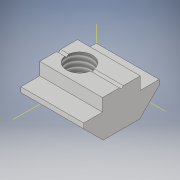
# Autodesk Inventor part: BTwnikel2_trajan20_21
Saved by Autodesk Inventor 2022.2 (Build 262287000, 287)
## iProperties
Company: HTBLA Kaindorf
RuleStatus: InUse
Created: 2022-06-22
Part Number: BTwnikel2_trajan20_21
Project: Zeichenmaschine_v2
Material: Generisch
Description: nutenstein
Document SubType Name: Modeling
Designer: trajan20
Density: 1 g/cm^3
Appearance: Vorgabe
Mass: 0.412179 g
Surface Area: 4.70943 cm^2
Volume: 0.412179 cm^3
AfterDocNew0: iProperties-Editor_aufrufen
Author: jan
Keywords: 2021
Autodesk Inventor part; units mm, degrees
ref_plane "YZ Plane" through (0, 0, 0) normal (1, 0, 0) x (0, 1, 0)
ref_plane "XZ Plane" through (0, 0, 0) normal (0, 1, 0) x (-1, 0, 0)
ref_plane "XY Plane" through (0, 0, 0) normal (0, 0, 1) x (1, 0, 0)
sketch "Skizze3" plane through (0, 0, 0) normal (0, 1, 0) x (-1, 0, 0)
  line L0 (0, 3.9) -> (-3, 3.9)
  line L1 (-3, 3.9) -> (-3, 5.9)
  line L2 (0, 3.9) -> (0, 3.1)
  line L3 (0, 3.1) -> (-3.1, 0)
  line L4 (-3, 5.9) -> (-5.7, 5.9)
  line L5 (-5.7, 5.9) -> (-6, 5.6)
  line L6 (-6, 5.6) -> (-6, 0)
  line L7 (-6, 0) -> (-3.1, 0)
  point P0 (0, 0)
  dimension "d6" = 3
  dimension "d7" = 6
  dimension "d8" = 3.1
  dimension "d9" = 5.9
  dimension "d10" = 135
  dimension "d11" = 0.3
  dimension "d12" = 2
  dimension "d13" = 135
  constraints: 16 end point, 3 perpendicular, 2 horizontal, 2 point on line, 1 vertical
  measures "d6" distance between parallel lines of L6 L1
  measures "d7" distance between parallel lines of L2 L6
  measures "d8" distance from line of L7 L2.end
  measures "d9" distance between parallel lines of L4 L7
  measures "d10" angle of L6 L5
  measures "d11" horizontal distance of L4.end L5.end
  measures "d12" distance between parallel lines of L4 L0
  measures "d13" angle of L3 L7
extrude "Extrusion3" add sketch "Skizze3" along normal blind 10
mirror "Spiegeln1" about plane through (6, 0, 5.6) normal (1, 0, 0) of "Extrusion3"
sketch "Skizze4" plane through (3.1, 0, 0) normal (0, 0, -1) x (-1, 0, 0)
  line L0 (0, 0) -> (0, 10) projected
  line L1 (-5.8, 0) -> (-5.8, 10) projected
  line L2 (-2.9, 0) -> (-2.9, 10) projected
  line L3 (0, 10) -> (-5.8, 10) projected
  line L4 (0, 0) -> (-5.8, 0) projected
  point P0 (3.1, 0)
  point P1 (-2.9, 3.3333)
  dimension "d23" = 10
  dimension "d24" = 3.3333
  constraints: 1 point on line
  measures "d23" distance between parallel lines of L3 L4
  measures "d24" distance from line of L4 point (-2.9, 3.333)
hole "Bohrung1" at (6, 3.3333, 0) direction (0, 0, 1) diameter 4.134 end through all thread size "M5x0.8" class "6H" standard "ISO Metric profile"
equation "\"d24\" = 0.333333 * d23"
